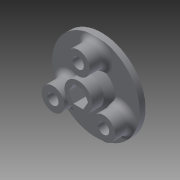
# Autodesk Inventor part: stick-holder-bottom
Saved by Autodesk Inventor 2014 (Build 180170000, 170)
## iProperties
Created: 2017-06-19
Part Number: stick-holder-bottom
Material: 一般
Document SubType Name: Modeling
Designer: hide
Density: 1 g/cm^3
Appearance: 既定
Author: hide
Autodesk Inventor part; units mm, degrees
ref_plane "YZ Plane" through (0, 0, 0) normal (1, 0, 0) x (0, 1, 0)
ref_plane "XZ Plane" through (0, 0, 0) normal (0, 1, 0) x (-1, 0, 0)
ref_plane "XY Plane" through (0, 0, 0) normal (0, 0, 1) x (1, 0, 0)
sketch "スケッチ1" plane through (0, 0, 0) normal (0, 1, 0) x (-1, 0, 0)
  circle A0 centre (0, 0) radius 1.75
  circle A1 centre (0, 0) radius 15
  circle A2 centre (0, 10) radius 1.9
  circle A3 centre (-8.6603, -5) radius 1.9
  circle A4 centre (8.6603, -5) radius 1.9
  dimension "d25" = 3.5
  dimension "d26" = 30
  dimension "d27" = 10
  dimension "d30" = 360
  dimension "d32" = 3.8
  constraints: 5 centre point, 2 coincident, 7 other
  measures "d25" diameter of A0
  measures "d26" diameter of A1
  measures "d27" distance of A2.centre point (0, 0)
  measures "d32" diameter of A2
extrude "押し出し1" add sketch "スケッチ1" along normal blind 2
sketch "スケッチ3" plane through (0, 0, 0) normal (0, 1, 0) x (-1, 0, 0)
  circle A0 centre (0, 0) radius 4.75
  dimension "d13" = 9.5
  constraints: 1 centre point, 1 coincident
  measures "d13" diameter of A0
extrude "押し出し2" add sketch "スケッチ3" against normal blind 7
sketch "スケッチ5" plane through (0, 0, 0) normal (0, 1, 0) x (-1, 0, 0)
  line L0 (-3.3486, 0) -> (-1.6743, 2.9)
  line L1 (-1.6743, 2.9) -> (1.6743, 2.9)
  line L2 (1.6743, 2.9) -> (3.3486, 0)
  line L3 (3.3486, 0) -> (1.6743, -2.9)
  line L4 (1.6743, -2.9) -> (-1.6743, -2.9)
  line L5 (-1.6743, -2.9) -> (-3.3486, 0)
  point P0 (0, 0)
  point P1 (0, 0)
  dimension "d18" = 5.8
  constraints: 12 end point, 1 coincident, 13 other
  measures "d18" distance between parallel lines of L4 L1
extrude "押し出し4" cut sketch "スケッチ5" against normal blind 7 and the other way blind 3.5
sketch "スケッチ6" plane through (0, 0, 0) normal (0, -1, 0) x (1, 0, 0)
  circle A0 centre (-8.6603, -5) radius 1.9 projected
  circle A1 centre (8.6603, -5) radius 1.9 projected
  circle A2 centre (0, 10) radius 1.9 projected
  circle A3 centre (0, 10) radius 3.9
  circle A4 centre (-8.6603, -5) radius 3.9
  circle A5 centre (8.6603, -5) radius 3.9
  dimension "d33" = 2
  dimension "d35" = 2
  dimension "d36" = 2
  constraints: 3 centre point, 3 coincident
  measures "d33" radial gap between concentric circles of A3 A2
  measures "d35" radial gap between concentric circles of A5 A1
  measures "d36" radial gap between concentric circles of A4 A0
extrude "押し出し5" add sketch "スケッチ6" along normal blind 6
sketch "スケッチ7" plane through (0, 2, 0) normal (0, 1, 0) x (1, 0, 0)
  circle A0 centre (0, -10) radius 1.9 projected
  circle A1 centre (8.6603, 5) radius 1.9 projected
  circle A2 centre (-8.6603, 5) radius 1.9 projected
extrude "押し出し6" add sketch "スケッチ7" against normal blind 1
chamfer "面取り2" distance 2 angle 45 1 edges at (4.75, 0, 0)
fillet "フィレット2" radius 2 6 edges at (-2.0448, 0, 13.321) (3.321, 0, 7.9552) (-4.7618, 0, -4.8897) (-12.0916, 0, -6.8537) (8.5499, 0, -8.8984) (10.5139, 0, -1.5687)
sketch "スケッチ8" plane through (0, -7, 0) normal (0, -1, 0) x (1, 0, 0)
  line L0 (3.3486, 0) -> (1.6743, -2.9) projected
  line L1 (1.6743, -2.9) -> (-1.6743, -2.9) projected
  line L2 (-1.6743, -2.9) -> (-3.3486, 0) projected
  line L3 (-3.3486, 0) -> (-1.6743, 2.9) projected
  line L4 (-1.6743, 2.9) -> (1.6743, 2.9) projected
  line L5 (1.6743, 2.9) -> (3.3486, 0) projected
  circle A0 centre (0, 0) radius 4.75 projected
  circle A1 centre (0, 0) radius 4.75
  constraints: 1 centre point, 1 coincident, 1 concentric
extrude "押し出し7" cut sketch "スケッチ8" against normal blind 1
equation "\"d35\" = d33"
equation "\"d36\" = d33"
